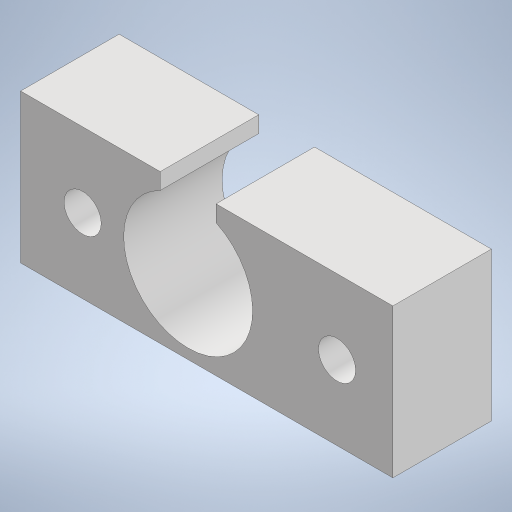
# Autodesk Inventor part: Pod
Saved by Autodesk Inventor 2023.2 (Build 272271000, 271)
## iProperties
Created: 2023-03-29
Part Number: Pod
Material: Generic
Document SubType Name: Modeling
Designer: Nathan Cai
Density: 1 g/cm^3
Appearance: Default
Author: Nathan Cai
Autodesk Inventor part; units mm, degrees
ref_plane "YZ Plane" through (0, 0, 0) normal (1, 0, 0) x (0, 1, 0)
ref_plane "XZ Plane" through (0, 0, 0) normal (0, 1, 0) x (-1, 0, 0)
ref_plane "XY Plane" through (0, 0, 0) normal (0, 0, 1) x (1, 0, 0)
sketch "Sketch1" plane through (0, 0, 0) normal (0, 0, 1) x (1, 0, 0)
  circle A0 centre (0, 0) radius 11
  line L0 (0, 0) -> (-18, 0) construction
  circle A1 centre (-18, 0) radius 3.175
  circle A2 centre (-18, 0) radius 38.1 construction
  circle A3 centre (25.4, 0) radius 1.7526 construction
  circle A4 centre (25.4, 0) radius 3.175
  line L1 (-28.575, 12.7) -> (34.925, 12.7)
  line L2 (34.925, 12.7) -> (34.925, -12.7)
  line L3 (34.925, -12.7) -> (-28.575, -12.7)
  line L4 (-28.575, -12.7) -> (-28.575, 12.7)
  line L5 (-28.575, 12.7) -> (34.925, -12.7) construction
  line L6 (34.925, 12.7) -> (-28.575, -12.7) construction
  point P0 (3.175, 0)
  dimension "d0" = 22
  dimension "d1" = 18
  dimension "d2" = 6.35
  dimension "d3" = 76.2
  dimension "d4" = 3.5052
  dimension "d5" = 25.4
  dimension "d6" = 6.35
  dimension "d7" = 63.5
  dimension "d8" = 25.4
  dimension "d9" = 3.175
  constraints: 14 end point, 5 centre point, 4 coincident, 2 horizontal, 2 midpoint, 2 parallel, 2 point on line, 1 perpendicular
  measures "d0" diameter of A0
  measures "d1" distance of L0.start L0.end
  measures "d2" diameter of A1
  measures "d3" diameter of A2
  measures "d4" diameter of A3
  measures "d5" distance of point (0, 0) A3.centre
  measures "d6" diameter of A4
  measures "d7" distance of L2.end L3.end
  measures "d8" distance of L1.end L2.end
  measures "d9" distance of point (0, 0) point (3.175, 0)
extrude "Extrusion1" add sketch "Sketch1" along normal blind 16.8
sketch "Sketch2" plane through (-28.575, 12.7, 0) normal (0, 1, 0) x (1, 0, 0)
  line L0 (0, -16.8) -> (63.5, -16.8) projected
  line L1 (31.75, -16.8) -> (31.75, 16.8) construction
  line L2 (28.575, -16.8) -> (28.575, 0) construction
  line L3 (0, 0) -> (63.5, 0) projected
  line L4 (33.3375, -16.8) -> (23.8125, -16.8)
  line L5 (23.8125, -16.8) -> (23.8125, 0)
  line L6 (23.8125, 0) -> (33.3375, 0)
  line L7 (33.3375, 0) -> (33.3375, -16.8)
  line L8 (33.3375, -16.8) -> (23.8125, 0) construction
  line L9 (23.8125, -16.8) -> (33.3375, 0) construction
  point P0 (28.575, 0)
  point P1 (63.5, 0)
  point P2 (31.75, 0)
  point P3 (28.575, -8.4)
  dimension "d12" = 3.175
  dimension "d13" = 9.525
  constraints: 16 end point, 5 midpoint, 2 parallel, 2 vertical, 1 horizontal, 1 perpendicular, 1 point on line, 4 other
  measures "d12" distance from line of point (31.75, 0) L2
  measures "d13" distance of L5.end L6.end
extrude "Extrusion2" cut sketch "Sketch2" against normal blind 19.05
body "Solid1"
